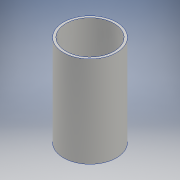
# Autodesk Inventor part: BearingHousing_Pipe
Saved by Autodesk Inventor 2018 (Build 220112000, 112)
## iProperties
Created: 2018-02-06
Part Number: BearingHousing_Pipe
Material: Aluminum 6061
Document SubType Name: Modeling
Designer: P136265
Density: 2.7 g/cm^3
Appearance: Aluminum - Flat
Author: P136265
Autodesk Inventor part; units mm, degrees
ref_plane "YZ Plane" through (0, 0, 0) normal (1, 0, 0) x (0, 1, 0)
ref_plane "XZ Plane" through (0, 0, 0) normal (0, 1, 0) x (-1, 0, 0)
ref_plane "XY Plane" through (0, 0, 0) normal (0, 0, 1) x (1, 0, 0)
sketch "Sketch1" plane through (0, 0, 0) normal (0, 0, 1) x (1, 0, 0)
  circle A0 centre (0, 0) radius 30.2
  circle A1 centre (0, 0) radius 27.5
  dimension "d0" = 60.4
  dimension "d4" = 2.7
  constraints: 2 centre point, 1 coincident
  measures "d0" diameter of A0
  measures "d4" radial gap between concentric circles of A0 A1
extrude "Extrusion2" add sketch "Sketch1" along normal blind 104
body "Solid2"
